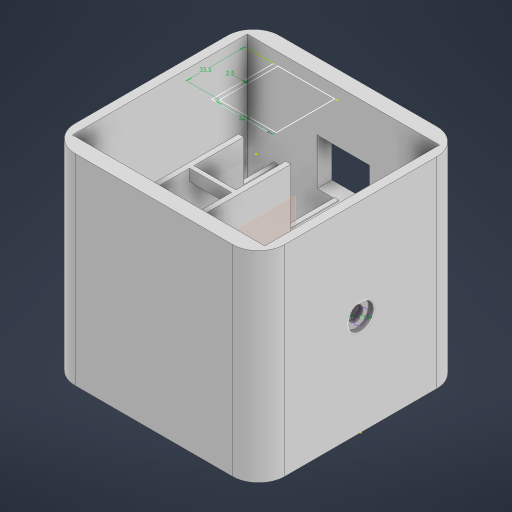
# Autodesk Inventor part: shooter-comp
Saved by Autodesk Inventor 2023 (Build 270158030, 158C)
## iProperties
Created: 2022-05-15
Part Number: shooter-comp
Material: Generic
Document SubType Name: Modeling
Designer: jayso
Density: 1 g/cm^3
Appearance: Default
Author: jayso
Autodesk Inventor part; units mm, degrees
ref_plane "YZ Plane" through (0, 0, 0) normal (1, 0, 0) x (0, 1, 0)
ref_plane "XZ Plane" through (0, 0, 0) normal (0, 1, 0) x (-1, 0, 0)
ref_plane "XY Plane" through (0, 0, 0) normal (0, 0, 1) x (1, 0, 0)
sketch "Sketch2" plane through (0, 0, 0) normal (0, 1, 0) x (-1, 0, 0)
  line L0 (60, 58.5) -> (-60, 58.5)
  line L1 (-60, 58.5) -> (-60, -58.5)
  line L2 (-60, -58.5) -> (60, -58.5)
  line L3 (60, -58.5) -> (60, 58.5)
  point P0 (0, 0)
  dimension "d0" = 117
  dimension "d1" = 120
  dimension "d2" = 58.5
  dimension "d3" = 60
  constraints: 8 end point, 2 parallel, 1 horizontal, 1 perpendicular
  measures "d0" distance between parallel lines of L2 L0
  measures "d1" distance of L1.end L2.end
  measures "d2" vertical distance of point (0, 0) L2.end
  measures "d3" horizontal distance of point (0, 0) L0.start
extrude "Extrusion1" add sketch "Sketch2" along normal blind 115
sketch "Sketch3" plane through (-60, 0, -58.5) normal (-1, 0, 0) x (0, 0, 1)
  circle A0 centre (58.5, 57.5) radius 4
  line L0 (0, 115) -> (117, 115) projected
  line L1 (0, 0) -> (0, 115) projected
  circle A1 centre (58.5, 57.5) radius 7.5
  point P0 (58.5, 0)
  point P1 (58.5, 115)
  dimension "d6" = 8
  dimension "d7" = 57.5
  dimension "d8" = 58.5
  dimension "d193" = 15
  constraints: 2 centre point, 1 coincident, 1 midpoint
  measures "d6" diameter of A0
  measures "d7" distance of point (58.5, 115) A0.centre
  measures "d8" distance from line of L1 A0.centre
  measures "d193" diameter of A1
sketch "Sketch4" plane through (0, 115, 0) normal (0, 1, 0) x (1, 0, 0)
  line L0 (-55, 50) -> (55, 50)
  line L1 (55, 50) -> (55, -50)
  line L2 (55, -50) -> (-55, -50)
  line L3 (-55, -50) -> (-55, 50)
  line L4 (-60, 58.5) -> (-60, -58.5) projected
  line L5 (-60, -58.5) -> (60, -58.5) projected
  point P0 (0, 0)
  dimension "d11" = 110
  dimension "d12" = 5
  dimension "d13" = 100
  dimension "d14" = 8.5
  constraints: 8 end point, 2 parallel, 1 horizontal, 1 perpendicular
  measures "d11" distance of L0.start L0.end
  measures "d12" distance between parallel lines of L4 L3
  measures "d13" distance of L0.end L1.end
  measures "d14" distance from line of L5 L1.end
extrude "Extrusion3" cut sketch "Sketch4" against normal blind 110
sketch "Sketch13" plane through (55, 115, 50) normal (0, 0, -1) x (-1, 0, 0)
  line L0 (40, -28) -> (70, -28)
  line L1 (70, -28) -> (70, -110)
  line L2 (70, -110) -> (40, -110)
  line L3 (40, -110) -> (40, -28)
  line L4 (0, 0) -> (110, 0) projected
  line L5 (0, -110) -> (110, -110) projected
  point P0 (55, -115)
  point P1 (55, 0)
  point P2 (70, -69)
  point P3 (40, -69)
  point P4 (55, -110)
  dimension "d44" = 28
  dimension "d45" = 40
  dimension "d46" = 40
  dimension "d47" = 0
  constraints: 8 end point, 4 midpoint, 2 parallel, 1 horizontal, 1 perpendicular
  measures "d44" distance from line of point (55, 0) L0
  measures "d45" horizontal distance of L4.end point (70, -69)
  measures "d46" horizontal distance of L4.start point (40, -69)
  measures "d47" distance from line of point (55, -110) L2
sketch "Sketch14" plane through (-55, 115, -50) normal (0, 0, 1) x (1, 0, 0)
  line L0 (0, -110) -> (110, -110) projected
  line L1 (40, -110) -> (70, -110)
  line L2 (70, -110) -> (70, -80)
  line L3 (70, -80) -> (40, -80)
  line L4 (40, -80) -> (40, -110)
  line L5 (0, 0) -> (0, -110) projected
  line L6 (110, 0) -> (110, -110) projected
  point P0 (55, -115)
  point P1 (40, -95)
  point P2 (70, -95)
  dimension "d48" = 40
  dimension "d49" = 40
  dimension "d50" = 30
  constraints: 8 end point, 2 midpoint, 2 parallel, 1 horizontal, 1 perpendicular, 1 point on line
  measures "d48" distance from line of L5 point (40, -95)
  measures "d49" distance from line of L6 point (70, -95)
  measures "d50" distance of L1.end L2.end
loft "Loft1" add profiles "Sketch13", "Sketch14"
sketch "Sketch18" plane through (-15, 5, 50) normal (-1, 0, 0) x (0, 0, 1)
  line L0 (-100, 0) -> (-100, 30) projected
  line L1 (-100, 0) -> (-55, 0)
  line L2 (0, 0) -> (-100, 0) projected
  line L3 (-55, 0) -> (-55, 53.4)
  line L4 (0, 82) -> (-100, 30) projected
  line L5 (-55, 53.4) -> (-105.2382, 30.2966)
  point P0 (-50, -5)
  dimension "d57" = 45
  constraints: 6 end point, 2 point on line, 1 perpendicular
  measures "d57" distance of L0.start L1.end
extrude "Extrusion7" cut sketch "Sketch18" against normal blind 30
ref_plane "Work Plane2" through (15, 5, 50) normal (1, 0, 0) x (0, 0, -1)
sketch "Sketch28" plane through (15, 5, 50) normal (1, 0, 0) x (0, 0, -1)
  line L0 (55, 0) -> (55, 53.4) projected
  line L1 (55, 53.4) -> (55, 118.4)
  line L2 (55, 53.4) -> (55, 0) projected
  line L3 (55, 118.4) -> (0, 118.4)
  line L4 (0, 82) -> (55, 53.4) projected
  line L5 (0, 118.4) -> (0, 82)
  line L6 (0, 82) -> (55, 53.4)
  point P0 (50, -5)
  dimension "d75" = 65
  constraints: 8 end point, 2 perpendicular, 1 collinear
  measures "d75" distance of L0.end L1.end
extrude "Extrusion8" add sketch "Sketch28" against normal blind 3
ref_plane "Work Plane3" through (-15, 5, 50) normal (-1, 0, 0) x (0, 0, 1)
sketch "Sketch31" plane through (-15, 5, 50) normal (-1, 0, 0) x (0, 0, 1)
  line L0 (0, 82) -> (-55, 53.4) projected
  line L1 (-55, 53.4) -> (-55, 117.6573)
  line L2 (-55, 0) -> (-55, 118.4) projected
  line L3 (-55, 118.4) -> (0, 118.4)
  line L4 (0, 118.4) -> (0, 82)
  point P0 (-50, -5)
  constraints: 6 end point, 1 horizontal, 1 perpendicular, 1 vertical
extrude "Extrusion9" add sketch "Sketch31" against normal blind 3
sketch "Sketch32" plane through (-15, 5, -5) normal (-1, 0, 0) x (0, 0, 1)
  line L0 (0, 0) -> (0, 118.4) projected
  line L1 (0, 118.4) -> (55, 118.4)
  line L2 (55, 118.4) -> (55, 103)
  line L3 (55, 103) -> (0, 103)
  line L4 (0, 103) -> (0, 118.4)
  point P0 (5, -5)
  point P1 (0, 103)
  dimension "d81" = 15.4
  constraints: 8 end point, 2 parallel, 1 horizontal, 1 perpendicular
  measures "d81" distance of L1.end L2.end
extrude "Extrusion10" cut sketch "Sketch32" against normal blind 30
sketch "Sketch43" plane through (60, 0, -58.5) normal (0, 0, -1) x (-1, 0, 0)
  line L0 (45, 5) -> (45, 108) projected
  line L1 (75, 108) -> (75, 5) projected
  line L2 (45, 85) -> (75, 85)
  line L3 (75, 85) -> (75, 58.4)
  line L4 (75, 58.4) -> (45, 58.4)
  line L5 (45, 58.4) -> (45, 85)
  line L6 (0, 115) -> (120, 115) projected
  line L7 (0, 0) -> (120, 0) projected
  point P0 (60, 0)
  point P1 (75, 85)
  point P2 (60, 115)
  point P3 (60, 85)
  point P4 (60, 0)
  dimension "d119" = 30
  dimension "d120" = 58.4
  constraints: 8 end point, 3 midpoint, 2 parallel, 2 point on line, 1 horizontal, 1 perpendicular
  measures "d119" distance of point (60, 115) point (60, 85)
  measures "d120" distance from line of point (60, 0) L4
extrude "Extrusion17" cut sketch "Sketch43" against normal blind 8.5
sketch "Sketch44" plane through (-15, 5, -5) normal (-1, 0, 0) x (0, 0, 1)
  line L0 (0, 103) -> (55, 103) projected
  line L1 (31, 91.6613) -> (0, 80)
  line L2 (0, 103) -> (0, 53.4) projected
  line L3 (55, 103) -> (55, 101)
  line L4 (31, 89.6613) -> (0, 78)
  line L5 (0, 78) -> (0, 80)
  line L6 (31, 91.6613) -> (31, 89.6613)
  point P0 (5, -5)
  dimension "d121" = 2
  dimension "d125" = 23
  dimension "d126" = 2
  constraints: 10 end point, 2 point on line, 2 vertical, 1 parallel
  measures "d121" distance of L0.end L3.end
  measures "d125" distance of L0.start L1.end
  measures "d126" distance of L1.end L4.end
extrude "Extrusion18" add sketch "Sketch44" against normal blind 30
sketch "Sketch46" plane through (12, 5, 50) normal (-1, 0, 0) x (0, 0, 1)
  line L0 (-55, 80) -> (-24, 91.6613) projected
  line L1 (-26.5, 90.7209) -> (-24, 91.6613)
  line L2 (-24, 91.6613) -> (-24, 103)
  line L3 (0, 103) -> (-55, 103) projected
  line L4 (-26.5, 103) -> (-26.5, 90.7209)
  point P0 (-50, -5)
  dimension "d127" = 2.5
  constraints: 6 end point, 3 point on line, 1 collinear, 1 parallel, 1 vertical
  measures "d127" distance between parallel lines of L2 L4
extrude "Extrusion19" add sketch "Sketch46" along normal blind 27
sketch "Sketch49" plane through (-12, 85, -5) normal (0, 0.935968, -0.352085) x (1, 0, 0)
  line L0 (0, -30.4498) -> (24, -30.4498) projected
  line L1 (24, -8.098) -> (24, 0) projected
  line L2 (0, -30.4498) -> (24, -30.4498)
  line L3 (24, -30.4498) -> (24, 0)
  line L4 (24, 0) -> (0, 0)
  line L5 (0, 0) -> (0, -30.4498)
  point P0 (12, 25.2474)
  point P1 (24, -30.4498)
  constraints: 8 end point, 2 parallel, 1 horizontal, 1 perpendicular
extrude "Extrusion21" cut sketch "Sketch49" against normal blind 3.5
sketch "Sketch50" plane through (15, 5, -5) normal (0, 0, -1) x (-1, 0, 0)
  line L0 (3, 82) -> (3, 53.4) projected
  line L1 (27, 53.4) -> (27, 82) projected
  line L2 (3, 78) -> (27, 78)
  line L3 (27, 78) -> (27, 80)
  line L4 (27, 80) -> (3, 80)
  line L5 (3, 80) -> (3, 78)
  line L6 (27, 80) -> (3, 80) projected
  line L7 (27, 78) -> (3, 78) projected
  point P0 (15, -5)
  point P1 (3, 80)
  point P2 (27, 78)
  dimension "d138" = 0
  dimension "d139" = 0
  constraints: 8 end point, 2 parallel, 2 point on line, 1 horizontal, 1 perpendicular
  measures "d138" distance between parallel lines of L6 L4
  measures "d139" distance between parallel lines of L7 L2
extrude "Extrusion22" cut sketch "Sketch50" against normal blind 1
sketch "Sketch51" plane through (12, 108, 23.5) normal (0, 0, -1) x (-1, 0, 0)
  line L0 (0, 0) -> (0, -13.3387) projected
  line L1 (24, -21) -> (24, 0) projected
  line L2 (0, -6.6693) -> (24, -6.6693)
  line L3 (24, -6.6693) -> (24, -14.1195)
  line L4 (24, -14.1195) -> (0, -14.1195)
  line L5 (0, -14.1195) -> (0, -6.6693)
  point P0 (12, -108)
  point P1 (24, -6.6693)
  constraints: 8 end point, 2 parallel, 1 horizontal, 1 midpoint, 1 perpendicular, 1 point on line
extrude "Extrusion23" cut sketch "Sketch51" against normal blind 3
sketch "Sketch54" plane through (15, 5, -5) normal (0, 0, -1) x (-1, 0, 0)
  line L0 (3, 53.4) -> (27, 53.4) projected
  line L1 (12.5, 53.4) -> (17.5, 53.4)
  line L2 (17.5, 53.4) -> (17.5, 0)
  line L3 (17.5, 0) -> (12.5, 0)
  line L4 (12.5, 0) -> (12.5, 53.4)
  line L5 (30, 103) -> (30, 0) projected
  line L6 (27, 53.4) -> (27, 103) projected
  line L7 (30, 0) -> (0, 0) projected
  point P0 (15, -5)
  point P1 (15, 0)
  point P2 (15, 0)
  dimension "d148" = 5
  dimension "d150" = 9.5
  dimension "d151" = 0
  constraints: 8 end point, 2 midpoint, 2 parallel, 1 horizontal, 1 perpendicular, 1 point on line
  measures "d148" distance of L2.end L3.end
  measures "d150" distance between parallel lines of L6 L2
  measures "d151" distance of point (15, 0) point (15, 0)
extrude "Extrusion25" add sketch "Sketch54" along normal blind 45
fillet "Face Fillet1" radius 10 1 edges at (0, 58.4, -5)
sketch "Sketch57" plane through (60, 0, 58.5) normal (1, 0, 0) x (0, 0, -1)
  circle A0 centre (58.5, 57.5) radius 4 projected
  circle A1 centre (58.5, 57.5) radius 4
  circle A2 centre (58.5, 57.5) radius 7.5
  point P0 (58.5, 0)
  dimension "d156" = 15
  constraints: 2 centre point, 2 coincident
  measures "d156" diameter of A2
extrude "Extrusion26" cut sketch "Sketch57" against normal blind 5 contours A0
extrude "Extrusion27" cut sketch "Sketch57" against normal blind 3
sketch "Sketch58" plane through (0, 5, 0) normal (0, 1, 0) x (1, 0, 0)
  line L0 (2.5, 50) -> (55, 50) projected
  line L1 (40, 50) -> (2.5, 50)
  line L2 (2.5, 50) -> (2.5, 14.5)
  line L3 (2.5, 14.5) -> (40, 14.5)
  line L4 (40, 14.5) -> (40, 50)
  line L5 (2.5, 7.4446) -> (2.5, 50) projected
  point P0 (0, 0)
  point P1 (2.5, 32.25)
  point P2 (2.5, 50)
  dimension "d161" = 35.5
  dimension "d162" = 37.5
  dimension "d163" = 0
  constraints: 8 end point, 2 parallel, 1 horizontal, 1 midpoint, 1 perpendicular, 1 point on line
  measures "d161" distance of L1.end L2.end
  measures "d162" distance of L2.end L3.end
  measures "d163" distance from line of L5 point (2.5, 32.25)
sketch "Sketch59" plane through (0, 5, 0) normal (0, 1, 0) x (1, 0, 0)
  line L0 (-2.5, 50) -> (-15, 50) projected
  line L1 (-2.5, 50) -> (-40, 50)
  line L2 (-40, 50) -> (-40, 14.5)
  line L3 (-40, 14.5) -> (-2.5, 14.5)
  line L4 (-2.5, 14.5) -> (-2.5, 50)
  line L5 (-2.5, 7.4446) -> (-2.5, 50) projected
  line L6 (-2.5, 14.5) -> (-40, 14.5)
  line L7 (-40, 14.5) -> (-40, 50)
  line L8 (-40, 50) -> (-2.5, 50)
  line L9 (-2.5, 50) -> (-2.5, 14.5)
  point P0 (0, 0)
  dimension "d164" = 37.5
  dimension "d165" = 35.5
  dimension "d166" = 0
  constraints: 16 end point, 4 parallel, 2 horizontal, 2 perpendicular, 1 point on line
  measures "d164" distance of L3.end L2.end
  measures "d165" distance of L1.end L2.end
  measures "d166" distance between parallel lines of L4 L5
extrude "Extrusion28" add sketch "Sketch58" along normal blind 103
sketch "Sketch60" plane through (0, 108, 0) normal (0, 1, 0) x (1, 0, 0)
  line L0 (-55, 50) -> (55, 50) projected
  line L1 (37.5, 16.5) -> (5, 16.5)
  line L2 (5, 16.5) -> (5, 50)
  line L3 (5, 50) -> (37.5, 50)
  line L4 (37.5, 50) -> (37.5, 16.5)
  line L5 (2.5, 50) -> (2.5, 14.5) projected
  line L6 (40, 14.5) -> (40, 50) projected
  line L7 (7.5, 14.5) -> (7.5, 50) projected
  line L8 (40, 14.5) -> (2.5, 14.5)
  line L9 (2.5, 14.5) -> (2.5, 50)
  line L10 (2.5, 50) -> (40, 50)
  line L11 (40, 50) -> (40, 14.5)
  point P0 (0, 0)
  point P1 (2.5, 14.5)
  dimension "d169" = 32.5
  dimension "d170" = 2.5
  dimension "d171" = 33.5
  constraints: 16 end point, 4 parallel, 2 horizontal, 2 perpendicular, 1 point on line
  measures "d169" distance of L1.start L1.end
  measures "d170" distance between parallel lines of L5 L2
  measures "d171" distance of L3.end L1.start
extrude "Extrusion29" add sketch "Sketch59" along normal blind 103
sketch "Sketch61" plane through (0, 108, 0) normal (0, 1, 0) x (1, 0, 0)
  line L0 (-40, 50) -> (-2.5, 50) projected
  line L1 (-5, 50) -> (-37.5, 50)
  line L2 (-37.5, 50) -> (-37.5, 16.5)
  line L3 (-37.5, 16.5) -> (-5, 16.5)
  line L4 (-5, 16.5) -> (-5, 50)
  line L5 (-40, 50) -> (-40, 14.5) projected
  line L6 (-55, 50) -> (-40, 50) projected
  line L7 (-7.5, 14.5) -> (-40, 14.5)
  line L8 (-40, 14.5) -> (-40, 50)
  line L9 (-40, 50) -> (-7.5, 50)
  point P0 (0, 0)
  point P1 (-40, 14.5)
  dimension "d174" = 32.5
  dimension "d175" = 33.5
  dimension "d176" = 2.5
  constraints: 14 end point, 3 parallel, 2 horizontal, 2 perpendicular, 1 point on line
  measures "d174" distance of L3.end L2.end
  measures "d175" distance of L1.end L2.end
  measures "d176" distance between parallel lines of L5 L2
extrude "Extrusion30" cut sketch "Sketch61" against normal blind 99
extrude "Extrusion32" cut sketch "Sketch60" against normal blind 99 contours L0 L7 L1 L2 | L0 L4 L1 L7
extrude "Extrusion33" cut sketch "Sketch60" against normal blind 49 contours L0 L2 L1 L7 L8 L5 | L7 L1 L4 L0 L6 L8
sketch "Sketch62" plane through (0, 9, 0) normal (0, 1, 0) x (1, 0, 0)
  line L0 (37.5, 50) -> (37.5, 16.5) projected
  line L1 (37.5, 16.5) -> (5, 16.5)
  line L2 (5, 16.5) -> (5, 21.5)
  line L3 (5, 21.5) -> (37.5, 21.5)
  line L4 (37.5, 21.5) -> (37.5, 16.5)
  point P0 (0, 0)
  dimension "d185" = 32.5
  dimension "d186" = 5
  constraints: 8 end point, 2 parallel, 1 horizontal, 1 perpendicular
  measures "d185" distance of L2.end L3.end
  measures "d186" distance of L1.end L2.end
extrude "Extrusion34" cut sketch "Sketch62" against normal blind 9
sketch "Sketch63" plane through (0, 9, 0) normal (0, 1, 0) x (1, 0, 0)
  line L0 (-5, 50) -> (-5, 16.5) projected
  line L1 (-5, 16.5) -> (-37.5, 16.5)
  line L2 (-37.5, 16.5) -> (-37.5, 21.5)
  line L3 (-37.5, 21.5) -> (-5, 21.5)
  line L4 (-5, 21.5) -> (-5, 16.5)
  point P0 (0, 0)
  point P1 (-5, 21.5)
  dimension "d189" = 32.5
  dimension "d190" = 5
  constraints: 8 end point, 2 parallel, 1 horizontal, 1 perpendicular
  measures "d189" distance of L2.end L3.end
  measures "d190" distance of L1.end L2.end
extrude "Extrusion35" cut sketch "Sketch63" against normal blind 9
extrude "Extrusion36" cut sketch "Sketch3" against normal blind 5 contours A0
extrude "Extrusion37" cut sketch "Sketch3" against normal blind 3
fillet "Face Fillet2" radius 15 1 edges at (-60, 57.5, -58.5)
fillet "Face Fillet3" radius 15 1 edges at (-60, 57.5, 58.5)
fillet "Face Fillet4" radius 15 1 edges at (60, 57.5, 58.5)
fillet "Face Fillet5" radius 15 1 edges at (60, 57.5, -58.5)
sketch "Sketch65" plane through (0, 108, 0) normal (0, 1, 0) x (1, 0, 0)
  line L0 (-2.5, 14.5) -> (-2.5, 50) projected
  line L1 (-2.5, 14.5) -> (-2.5, 50)
  line L2 (-5, 50) -> (-2.5, 50) projected
  line L3 (-2.5, 50) -> (-5, 50)
  line L4 (-5, 16.5) -> (-5, 21.5) projected
  line L5 (-5, 50) -> (-5, 16.5)
  line L6 (-37.5, 16.5) -> (-5, 16.5) projected
  line L7 (-5, 16.5) -> (-37.5, 16.5)
  line L8 (-37.5, 16.5) -> (-37.5, 50)
  line L9 (-55, 50) -> (55, 50) projected
  line L10 (-40, 50) -> (-40, 14.5) projected
  line L11 (-40, 50) -> (-40, 14.5)
  line L12 (-2.5, 5) -> (-2.5, 14.5) projected
  line L13 (-40, 14.5) -> (-2.5, 14.5)
  point P0 (0, 0)
  constraints: 14 end point, 4 collinear, 2 perpendicular, 1 point on line, 1 vertical
extrude "Extrusion38" cut sketch "Sketch65" against normal blind 49 contours L13 L10 L9 L8 L6 L4 L5 L2 L0
body "Solid1"
